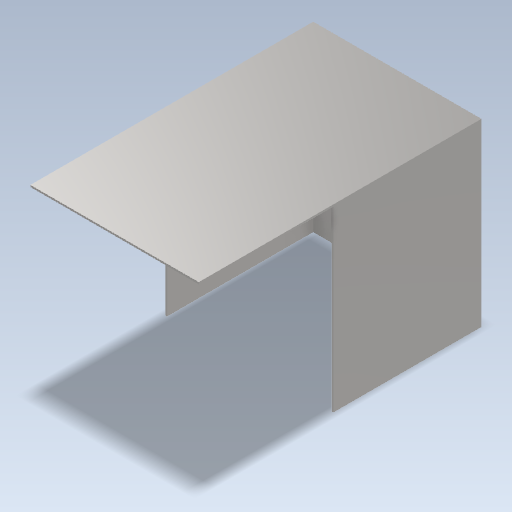
# Autodesk Inventor part: Pump System Cover
Saved by Autodesk Inventor 2020 (Build 240168000, 168)
## iProperties
Created: 2020-08-16
Part Number: Pump System Cover
Material: Generic
Document SubType Name: Modeling
Designer: Abbas
Density: 1 g/cm^3
Appearance: Default
Author: Abbas
Autodesk Inventor part; units mm, degrees
ref_plane "YZ Plane" through (0, 0, 0) normal (1, 0, 0) x (0, 1, 0)
ref_plane "XZ Plane" through (0, 0, 0) normal (0, 1, 0) x (-1, 0, 0)
ref_plane "XY Plane" through (0, 0, 0) normal (0, 0, 1) x (1, 0, 0)
sketch "Sketch1" plane through (0, 0, 0) normal (1, 0, 0) x (0, 1, 0)
  line L0 (0, 0) -> (0, -200)
  line L1 (0, 0) -> (200, 0) construction
  line L2 (0, -200) -> (-240, -200)
  line L3 (-240, -420) -> (0, -420)
  line L4 (0, 0) -> (3, 0)
  line L5 (3, 0) -> (3, -420)
  line L6 (3, -420) -> (-1.1181, -420)
  line L7 (0, -200) -> (0, -420)
  line L8 (-240, -417) -> (0, -417)
  line L9 (-240, -417) -> (0, -417) construction
  line L10 (-240, -200) -> (-265, -200)
  line L11 (-265, -200) -> (-265, -420)
  line L12 (-265, -420) -> (-240, -420)
  line L13 (-240, -417) -> (-265, -417)
  dimension "d0" = 200
  dimension "d1" = 90
  dimension "d2" = 240
  dimension "d3" = 90
  dimension "d4" = 220
  dimension "d8" = 3
  dimension "d9" = 90
  dimension "d10" = 3
  dimension "d18" = 25
  dimension "d19" = 220
  dimension "d20" = 90
  constraints: 28 end point, 5 point on line, 4 horizontal, 2 equal length, 2 perpendicular, 2 vertical
  measures "d0" distance of L0.start L0.end
  measures "d1" angle of L0 L1
  measures "d2" distance of L0.end L2.end
  measures "d3" angle of L0 L2
  measures "d4" distance of L2.end L3.start
  measures "d8" distance of L0.start L4.end
  measures "d9" angle of L4 L5
  measures "d10" distance of L8.start L3.start
  measures "d18" distance of L2.end L10.end
  measures "d19" distance of L10.end L11.end
  measures "d20" angle of L11 L10
extrude "Extrusion4" add sketch "Sketch1" against normal blind 250 contours L4 L5 L6 L7 L0 | L7 L3 L12 L11 L13 L8
extrude "Extrusion5" add sketch "Sketch1" against normal blind 3 contours L7 L8 L13 L11 L10 L2
sketch "Sketch3" plane through (-250, 0, 0) normal (-1, 0, 0) x (0, 0, 1)
  line L0 (-417, -265) -> (-417, 0) projected
  line L1 (-200, -265) -> (-200, 0) projected
  line L2 (-417, 0) -> (-200, 0)
  line L3 (-417, -265) -> (-200, -265) projected
  line L4 (-200, 0) -> (-200, -265)
  line L5 (-200, -265) -> (-417, -265)
  point P0 (0, 0)
  constraints: 6 end point, 2 perpendicular, 1 collinear
extrude "Extrusion6" add sketch "Sketch3" against normal blind 3
body "Solid2"
